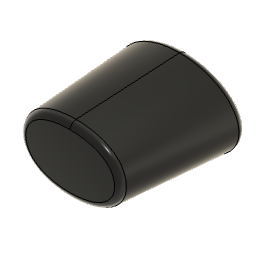
sharpener-f3d (Autodesk Fusion 360 design; units mm, degrees)
Autodesk Fusion 360 part; units mm, degrees
sketch "Topdown" plane through (0, 0, 0) normal (0, 0, 1) x (1, 0, 0)
  line L0 (0, 0) -> (0, 37.6) construction
  line L1 (-19.55, 37.6) -> (19.55, 37.6)
  line L2 (-16.25, 0) -> (16.25, 0)
  dimension "d1" = 37.6
  dimension "d4" = 39.1
  dimension "d5" = 32.5
  constraint coincident L0.start origin
  constraint vertical L0
  constraint horizontal L1
  constraint midpoint L0.end L1
  constraint horizontal L2
  constraint midpoint L0.start L2
  measures "d1" distance of L0.start L0.end
  measures "d4" distance of L1.start L1.end
  measures "d5" distance of L2.start L2.end
sketch "Sideview" plane through (0, 0, 0) normal (1, 0, 0) x (0, 1, 0)
  line L0 (0, 0) -> (37.6, 0)
  line L1 (0, 10.75) -> (0, -10.75)
  line L2 (37.6, 12.85) -> (37.6, -12.85)
  point P0 (37.6, 0)
  dimension "d7" = 21.5
  dimension "d8" = 25.7
  constraint vertical L1
  constraint midpoint L1 L0.start
  constraint vertical L2
  constraint midpoint L2 P0
  measures "d7" distance of L1.start L1.end
  measures "d8" distance of L2.start L2.end
sketch "Front-view" plane through (0, 0, 0) normal (0, 1, 0) x (1, 0, 0)
  spline S0 degree 5 poles (0, -10.75) (1.1627, -10.7456) (3.488, -10.629) (6.8659, -10.132) (10.7094, -8.8558) (14.0969, -6.4111) (15.9993, -3.3621) (16.56, 0.0002) (15.8867, 3.3617) (13.909, 6.4092) (10.5126, 8.8528) (5.7747, 10.4485) (0, 11.0239) (-5.7747, 10.4994) (-10.5126, 8.9289) (-13.909, 6.4809) (-15.8867, 3.4039) (-16.56, -0.0002) (-15.9993, -3.4035) (-14.0969, -6.4789) (-10.7094, -8.9258) (-6.8659, -10.1826) (-3.488, -10.6554) (-1.1627, -10.7544) (0, -10.75) knots 0 0 0 0 0 0 0.05 0.1 0.15 0.2 0.25 0.3 0.35 0.4 0.45 0.5 0.55 0.6 0.65 0.7 0.75 0.8 0.85 0.9 0.95 1 1 1 1 1 1
  line L0 (-5.4804, -10.7707) -> (5.4804, -10.7293)
  line L1 (5.3574, 10.727) -> (-5.3574, 10.773)
  point P0 (0, -10.75)
  point P1 (16.25, 0)
  point P2 (0, 10.75)
  point P3 (-16.25, 0)
  point P4 (16.25, 0)
  point P5 (0, 10.75)
  point P6 (-16.25, 0)
  constraint coincident P0 S0.start
  constraint coincident P4 P1
  constraint coincident P5 P2
  constraint coincident P6 P3
  constraint midpoint P0 L0
  constraint midpoint P5 L1
ref_plane "WorkPlane1" through (0, 37.6, 0) normal (0, 1, 0) x (0, 0, 1)
sketch "Back-view" plane through (0, 37.6, 0) normal (0, 1, 0) x (1, 0, 0)
  spline S0 degree 5 poles (0, -12.85) (1.2207, -12.85) (3.662, -12.7212) (7.2657, -12.1415) (11.721, -10.6277) (16.1689, -7.7041) (19.0479, -4.0436) (20.048, 0) (19.0479, 4.0436) (16.1689, 7.7041) (11.721, 10.6277) (6.1519, 12.52) (0, 13.1774) (-6.1519, 12.52) (-11.721, 10.6277) (-16.1689, 7.7041) (-19.0479, 4.0436) (-20.048, 0) (-19.0479, -4.0436) (-16.1689, -7.7041) (-11.721, -10.6277) (-7.2657, -12.1415) (-3.662, -12.7212) (-1.2207, -12.85) (0, -12.85) knots 0 0 0 0 0 0 0.05 0.1 0.15 0.2 0.25 0.3 0.35 0.4 0.45 0.5 0.55 0.6 0.65 0.7 0.75 0.8 0.85 0.9 0.95 1 1 1 1 1 1
  line L0 (0, 0) -> (-19.55, 0) construction
  line L1 (0, 0) -> (19.55, 0) construction
  circle A0 centre (9.775, 0) radius 5.65
  circle A1 centre (-9.775, 0) radius 4.05
  point P0 (19.55, 0)
  point P1 (0, -12.85)
  point P2 (-19.55, 0)
  point P3 (0, 12.85)
  point P4 (19.55, 0)
  point P5 (0, 12.85)
  point P6 (-19.55, 0)
  dimension "d10" = 11.3
  dimension "d11" = 8.1
  constraint coincident P6 P2
  constraint coincident P1 S0.start
  constraint coincident L0.start L1.start
  constraint coincident P4 P0
  constraint midpoint L1 A0.centre
  constraint midpoint L0 A1.centre
  measures "d10" diameter of A0
  measures "d11" diameter of A1
loft "Loft1" add profiles "Back-view", "Front-view" section 1 contours S0 | A0 | A1 section 2
ref_plane "WorkPlane2" through (0, 22.6, 0) normal (0, 1, 0) x (0, 0, 1)
sketch "Sketch5" plane through (0, 22.6, 0) normal (0, 1, 0) x (1, 0, 0)
  circle A0 centre (-9.775, 0) radius 4.05
  circle A1 centre (9.775, 0) radius 5.65
  circle A2 centre (9.775, 0) radius 1.65
  circle A3 centre (-9.775, 0) radius 1.55
  dimension "d13" = -4
  dimension "d14" = -2.5
loft "Loft2" cut profiles "Back-view", "Sketch5" section 1 contours A0 section 2 contours A2
loft "Loft3" cut profiles "Back-view", "Sketch5" section 1 contours A1 section 2 contours A3
fillet "Fillet1" radius 1.5 1 faces at (-8.9356, 35.9333, 3.6776)
fillet "Fillet2" radius 1.5 1 faces at (9.386, 35.9333, -5.191)
fillet "Fillet3" radius 2 1 edges at (0, 37.6, -12.85)
fillet "Fillet4" radius 2 1 edges at (0, 0, -10.75)
